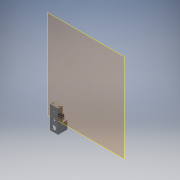
# Autodesk Inventor part: Xendmotorside
Saved by Autodesk Inventor 2016 (Build 200138000, 138)
## iProperties
Created: 2016-05-27
Part Number: Xendmotorside
Material: Generic
Document SubType Name: Modeling
Designer: Scott
Density: 1 g/cm^3
Appearance: Default
Author: Scott
Autodesk Inventor part; units mm, degrees
ref_plane "YZ Plane" through (0, 0, 0) normal (1, 0, 0) x (0, 1, 0)
ref_plane "XZ Plane" through (0, 0, 0) normal (0, 1, 0) x (-1, 0, 0)
ref_plane "XY Plane" through (0, 0, 0) normal (0, 0, 1) x (1, 0, 0)
ref_plane "Work Plane1" through (0, 0, 0) normal (0, 0, 1) x (1, 0, 0)
sketch "Sketch1" plane through (0, 0, 0) normal (0, 0, 1) x (1, 0, 0)
  circle A0 centre (0, 0) radius 6.35 projected
  circle A1 centre (0.5752, -49.1016) radius 4 projected
  line L0 (-12.7, -22.86) -> (12.7, -22.86)
  line L1 (12.7, -22.86) -> (12.7, 22.86)
  line L2 (12.7, 22.86) -> (-12.7, 22.86)
  line L3 (-12.7, 22.86) -> (-12.7, -22.86)
  line L4 (-12.7, -22.86) -> (12.7, 22.86) construction
  line L5 (12.7, -22.86) -> (-12.7, 22.86) construction
  line L6 (12.7, 22.86) -> (-12.7, 22.86)
  line L7 (-12.7, 22.86) -> (-12.7, -66.04)
  line L8 (-12.7, -66.04) -> (12.7, -66.04)
  line L9 (12.7, -66.04) -> (12.7, 22.86)
  point P0 (0, 0)
  dimension "d0" = 25.4
  dimension "d1" = 45.72
  dimension "d2" = 88.9
  constraints: 20 end point, 4 parallel, 2 horizontal, 2 midpoint, 2 perpendicular
  measures "d0" distance of L2.end L1.end
  measures "d1" distance of L1.end L0.end
  measures "d2" distance of L7.end L6.end
extrude "Extrusion1" add sketch "Sketch1" along normal blind 2.54
sketch "Sketch2" plane through (0, 0, 2.54) normal (0, 0, 1) x (1, 0, 0)
  circle A0 centre (0, 0) radius 6.35 projected
  circle A1 centre (0.5752, -49.1016) radius 4 projected
  line L0 (12.7, 22.86) -> (-12.7, 22.86) projected
  line L1 (-12.7, 22.86) -> (-12.7, -66.04) projected
  line L2 (-12.7, -66.04) -> (12.7, -66.04) projected
  line L3 (12.7, -66.04) -> (12.7, 22.86) projected
  circle A2 centre (0, 0) radius 7.62
  line L4 (0, 0) -> (0, -12.7)
  circle A3 centre (0, -12.7) radius 2.54
  line L5 (0, 0) -> (0, 12.7)
  circle A4 centre (0, 12.7) radius 2.54
  circle A5 centre (0.5752, -49.1016) radius 4 projected
  circle A6 centre (0.5752, -49.1016) radius 5
  point P0 (0, 0)
  dimension "d5" = 15.24
  dimension "d6" = 12.7
  dimension "d7" = 5.08
  dimension "d8" = 12.7
  dimension "d9" = 5.08
  dimension "d10" = 10
  constraints: 4 centre point, 4 coincident, 4 end point, 2 vertical
  measures "d5" diameter of A2
  measures "d6" distance of L4.start L4.end
  measures "d7" diameter of A3
  measures "d8" distance of L4.start L5.end
  measures "d9" diameter of A4
  measures "d10" diameter of A6
extrude "Extrusion2" cut sketch "Sketch2" against normal blind 2.54 contours A0 L4 L5 | A0 L5 A2 L4 | L5 L4 A0 | A0 L4 A2 L5 | A3 | A4 | A6
sketch "Sketch3" plane through (0, 0, 0) normal (0, 0, -1) x (-1, 0, 0)
  circle A0 centre (0, 0) radius 7.62 projected
  circle A1 centre (0, 12.7) radius 2.54 projected
  circle A2 centre (0, -12.7) radius 2.54 projected
  circle A3 centre (-0.5752, -49.1016) radius 5 projected
  line L0 (-12.7, 22.86) -> (12.7, 22.86) projected
  line L1 (-12.7, -66.04) -> (-12.7, 22.86) projected
  line L2 (12.7, -66.04) -> (-12.7, -66.04) projected
  line L3 (12.7, 22.86) -> (12.7, -66.04) projected
  line L4 (10.16, 19.05) -> (-10.16, 19.05)
  line L5 (-10.16, 19.05) -> (-10.16, -19.05)
  line L6 (-10.16, -19.05) -> (10.16, -19.05)
  line L7 (10.16, -19.05) -> (10.16, 19.05)
  circle A4 centre (0, 0) radius 7.62 projected
  line L8 (10.16, 19.05) -> (-10.16, -19.05) construction
  line L9 (-10.16, 19.05) -> (10.16, -19.05) construction
  point P0 (0, 0)
  dimension "d13" = 20.32
  dimension "d14" = 38.1
  constraints: 12 end point, 2 midpoint, 2 parallel, 1 horizontal, 1 perpendicular
  measures "d13" distance of L6.end L5.end
  measures "d14" distance of L5.end L4.end
extrude "Extrusion3" add sketch "Sketch3" along normal blind 25.4 contours L0 L3 L2 L1
sketch "Sketch4" plane through (0, 0, 2.54) normal (0, 0, 1) x (1, 0, 0)
  line L0 (-12.7, -66.04) -> (12.7, -66.04) projected
  line L1 (0, -66.04) -> (0, -90.8431)
  line L2 (24.81, -115.6589) -> (-24.81, -115.6589)
  line L3 (-24.81, -115.6589) -> (-24.81, -66.0273)
  line L4 (-24.81, -66.0273) -> (24.81, -66.0273)
  line L5 (24.81, -66.0273) -> (24.81, -115.6589)
  line L6 (24.81, -115.6589) -> (-24.81, -66.0273) construction
  line L7 (-24.81, -115.6589) -> (24.81, -66.0273) construction
  circle A0 centre (0, -90.8431) radius 12.5
  line L8 (0, -90.8431) -> (-15.5, -90.8431)
  line L9 (-15.5, -90.8431) -> (-15.5, -75.3431)
  circle A1 centre (-15.5, -75.3431) radius 2
  circle A2 centre (-15.5, -106.3467) radius 2
  circle A3 centre (15.5, -106.3467) radius 2
  circle A4 centre (15.5, -75.3395) radius 2
  point P0 (0, 0)
  dimension "d17" = 24.8031
  dimension "d18" = 49.62
  dimension "d19" = 49.6316
  dimension "d20" = 25
  dimension "d21" = 15.5
  dimension "d22" = 15.5
  dimension "d23" = 4
  dimension "d24" = 4
  dimension "d25" = 4
  dimension "d26" = 4
  constraints: 18 end point, 5 centre point, 3 midpoint, 3 point on line, 2 coincident, 2 horizontal, 2 parallel, 2 vertical, 1 perpendicular
  measures "d17" distance of L1.start L1.end
  measures "d18" distance of L3.end L4.end
  measures "d19" distance of L2.end L3.end
  measures "d20" diameter of A0
  measures "d21" distance of L8.start L8.end
  measures "d22" distance of L8.end L9.end
  measures "d23" diameter of A1
  measures "d24" diameter of A2
  measures "d25" diameter of A3
  measures "d26" diameter of A4
extrude "Extrusion4" add sketch "Sketch4" against normal blind 5.08
sketch "Sketch5" plane through (0, 0, -2.54) normal (0, 0, -1) x (-1, 0, 0)
  circle A0 centre (0, -90.8431) radius 12.5 projected
  circle A1 centre (-15.5, -75.3395) radius 2 projected
  circle A2 centre (-15.5, -106.3467) radius 2 projected
  circle A3 centre (15.5, -106.3467) radius 2 projected
  circle A4 centre (15.5, -75.3431) radius 2 projected
  line L0 (-12.7, -66.0273) -> (-12.7, 22.86) projected
  line L1 (-12.7, 22.86) -> (12.7, 22.86) projected
  line L2 (12.7, 22.86) -> (12.7, -66.0273) projected
  line L3 (24.81, -66.0273) -> (12.7, -66.0273) projected
  line L4 (24.81, -115.6589) -> (24.81, -66.0273) projected
  line L5 (-24.81, -115.6589) -> (24.81, -115.6589) projected
  line L6 (-24.81, -66.0273) -> (-24.81, -115.6589) projected
  line L7 (-12.7, -66.0273) -> (-24.81, -66.0273) projected
  circle A5 centre (0, 0) radius 7.62 projected
  circle A6 centre (0, 12.7) radius 2.54 projected
  circle A7 centre (0, -12.7) radius 2.54 projected
  circle A8 centre (-0.5752, -49.1016) radius 5 projected
  line L8 (24.81, -66.0273) -> (12.7, -66.0273) projected
  line L9 (-24.81, -115.6589) -> (24.81, -115.6589)
  line L10 (24.81, -115.6589) -> (24.81, -66.0273)
  line L11 (24.81, -66.0273) -> (-24.81, -66.0273)
  line L12 (-24.81, -66.0273) -> (-24.81, -115.6589)
  line L13 (-24.81, -115.6589) -> (24.81, -66.0273) construction
  line L14 (24.81, -115.6589) -> (-24.81, -66.0273) construction
  line L15 (-22, -112.8431) -> (22, -112.8431)
  line L16 (22, -112.8431) -> (22, -68.8431)
  line L17 (22, -68.8431) -> (-22, -68.8431)
  line L18 (-22, -68.8431) -> (-22, -112.8431)
  line L19 (-22, -112.8431) -> (22, -68.8431) construction
  line L20 (22, -112.8431) -> (-22, -68.8431) construction
  point P0 (0, 0)
  dimension "d29" = 44
  dimension "d30" = 44
  constraints: 24 end point, 4 midpoint, 4 parallel, 2 horizontal, 2 perpendicular
  measures "d29" distance of L17.end L16.end
  measures "d30" distance of L16.end L15.end
extrude "Extrusion5" add sketch "Sketch5" along normal blind 50.8 contours L11 L3 L4 L5 L6 L7
sketch "Sketch6" plane through (0, 0, -53.34) normal (0, 0, -1) x (-1, 0, 0)
  line L0 (22, -68.8431) -> (22, -112.8431) projected
  line L1 (22, -112.8431) -> (50.6459, -112.8431)
  line L2 (50.6459, -112.8431) -> (50.6459, -68.8431)
  line L3 (50.6459, -68.8431) -> (22, -68.8431)
  line L4 (22, -68.8431) -> (22, -112.8431)
  point P0 (0, 0)
  constraints: 8 end point, 2 parallel, 1 horizontal, 1 perpendicular
extrude "Extrusion6" cut sketch "Sketch6" against normal blind 50.8
chamfer "Chamfer1" distance 44.45 angle 45 1 edges at (-24.81, -114.251, -53.34)
sketch "Sketch7" plane through (12.7, -66.0273, 2.54) normal (0, 1, 0) x (1, 0, 0)
  line L0 (-25.4, 27.94) -> (-25.4, 0) projected
  line L1 (0, 27.94) -> (-25.4, 27.94) projected
  line L2 (0, 0) -> (0, 27.94) projected
  line L3 (0, 0) -> (12.11, 0) projected
  line L4 (12.11, 0) -> (12.11, 55.88) projected
  line L5 (-37.51, 55.88) -> (12.11, 55.88) projected
  line L6 (-37.51, 0) -> (-37.51, 55.88) projected
  line L7 (-37.51, 0) -> (-25.4, 0) projected
  line L8 (6.055, 0) -> (6.055, 12.7)
  circle A0 centre (6.055, 12.7) radius 4
  circle A1 centre (-31.455, 12.7) radius 4
  line L9 (0, 27.94) -> (12.11, 27.94)
  line L10 (12.11, 0) -> (12.11, 55.88) projected
  line L11 (-25.4, 27.94) -> (-37.51, 27.94)
  line L12 (-37.51, 55.88) -> (-37.51, 5.08) projected
  point P0 (-12.7, 2.54)
  dimension "d38" = 12.7
  dimension "d39" = 8
  dimension "d40" = 8
  constraints: 6 end point, 2 centre point, 2 midpoint, 2 point on line, 1 coincident, 1 vertical
  measures "d38" distance of L8.start L8.end
  measures "d39" diameter of A0
  measures "d40" diameter of A1
extrude "Extrusion7" add sketch "Sketch7" along normal up to surface (88.8873 mm away) contours L0 L7 L6 L11 | L9 L4 L3 L2
sketch "Sketch8" plane through (0, 0, -25.4) normal (0, 0, -1) x (-1, 0, 0)
  line L0 (24.81, -66.0273) -> (-24.81, -66.0273) projected
  line L1 (24.81, -66.0273) -> (24.81, 22.86) projected
  line L2 (24.81, 22.86) -> (-24.81, 22.86) projected
  line L3 (-24.81, -66.0273) -> (-24.81, 22.86) projected
  line L4 (10.16, 19.05) -> (10.16, -19.05) projected
  line L5 (10.16, -19.05) -> (-10.16, -19.05) projected
  line L6 (-10.16, -19.05) -> (-10.16, 19.05) projected
  line L7 (-10.16, 19.05) -> (10.16, 19.05) projected
  circle A0 centre (-0.5752, -49.1016) radius 5 projected
  circle A1 centre (-0.5752, -49.1016) radius 12.7
  point P0 (0, 0)
  dimension "d43" = 25.4
  constraints: 1 centre point, 1 coincident
  measures "d43" diameter of A1
extrude "Extrusion8" add sketch "Sketch8" along normal blind 12.7 contours A1
sketch "Sketch9" plane through (0.5752, -49.1016, -38.1) normal (0, 0, -1) x (-1, 0, 0)
  circle A0 centre (0, 0) radius 12.7 projected
  line L0 (25.3852, -16.9257) -> (-24.2348, -16.9257) projected
  line L1 (25.3852, -16.9257) -> (25.3852, 71.9616) projected
  line L2 (25.3852, 71.9616) -> (-24.2348, 71.9616) projected
  line L3 (-24.2348, -16.9257) -> (-24.2348, 71.9616) projected
  line L4 (10.7352, 68.1516) -> (10.7352, 30.0516) projected
  line L5 (10.7352, 30.0516) -> (-9.5848, 30.0516) projected
  line L6 (-9.5848, 30.0516) -> (-9.5848, 68.1516) projected
  line L7 (-9.5848, 68.1516) -> (10.7352, 68.1516) projected
  line L8 (-12.7, 0) -> (-12.7, -16.9257)
  line L9 (25.3852, -16.9257) -> (-24.2348, -16.9257) projected
  circle A1 centre (0, 0) radius 12.7 projected
  line L10 (12.7, 0) -> (12.7, -16.9257)
  line L11 (12.7, -16.9257) -> (-12.7, -16.9257)
  point P0 (0.5752, 49.1016)
  constraints: 6 end point, 2 perpendicular, 2 point on circle, 2 point on line, 1 collinear, 1 horizontal alignment, 1 vertical, 1 other
extrude "Extrusion9" add sketch "Sketch9" against normal up to surface (12.7 mm away) contours L10 L0 L8 A0
sketch "Sketch10" plane through (0, 0, -38.1) normal (0, 0, -1) x (-1, 0, 0)
  circle A0 centre (-0.5752, -49.1016) radius 5 projected
  circle A1 centre (-0.5752, -49.1016) radius 7.5
  point P0 (0, 0)
  dimension "d48" = 15
  constraints: 1 centre point, 1 coincident
  measures "d48" diameter of A1
sketch "Sketch11" plane through (0, 0, 2.54) normal (0, 0, 1) x (1, 0, 0)
  circle A0 centre (0.5752, -49.1016) radius 5 projected
  circle A1 centre (0.5752, -49.1016) radius 7.5
  point P0 (0, 0)
  dimension "d49" = 15
  constraints: 1 centre point, 1 coincident
  measures "d49" diameter of A1
extrude "Extrusion10" cut sketch "Sketch11" against normal blind 24
sketch "Sketch12" plane through (0, 0, -38.1) normal (0, 0, -1) x (-1, 0, 0)
  circle A0 centre (-0.5752, -49.1016) radius 5 projected
  arc A1 (12.1248, -49.1016) -> (-13.2752, -49.1016) centre (-0.5752, -49.1016) ccw projected
  line L0 (-13.2752, -49.1016) -> (-13.2752, -66.0273) projected
  line L1 (12.1248, -66.0273) -> (-13.2752, -66.0273) projected
  line L2 (12.1248, -66.0273) -> (12.1248, -49.1016) projected
  point P0 (0, 0)
extrude "Extrusion11" add sketch "Sketch12" along normal blind 8.89
sketch "Sketch13" plane through (0, 0, -46.99) normal (0, 0, -1) x (-1, 0, 0)
  circle A0 centre (-0.5752, -49.1016) radius 5 projected
  arc A1 (12.1248, -49.1016) -> (-13.2752, -49.1016) centre (-0.5752, -49.1016) ccw projected
  line L0 (-13.2752, -49.1016) -> (-13.2752, -66.0273) projected
  line L1 (12.1248, -66.0273) -> (-13.2752, -66.0273) projected
  line L2 (12.1248, -66.0273) -> (12.1248, -49.1016) projected
  circle A2 centre (-0.5752, -49.1016) radius 7.5
  point P0 (0, 0)
  dimension "d54" = 15
  constraints: 1 centre point, 1 coincident
  measures "d54" diameter of A2
extrude "Extrusion12" cut sketch "Sketch13" against normal blind 24 contours A2
sketch "Sketch14" plane through (24.81, -115.6589, 2.54) normal (1, 0, 0) x (0, 0, -1)
  spline S0 degree 2 poles (6.6012, 5.0914) (10.3495, 6.6696) (13.0128, 10.9605) knots 0 0 0 1 1 1
  spline S1 degree 2 poles (13.0128, 10.9605) (14.6897, 14.0677) (14.6897, 14.6102) knots 0 0 0 1 1 1
  line L0 (14.6897, 14.6102) -> (14.2952, 14.6102)
  spline S2 degree 2 poles (14.2952, 14.6102) (13.0128, 14.6102) (8.8206, 7.0642) knots 0 0 0 1 1 1
  line L1 (8.8206, 7.0642) -> (8.722, 7.0642)
  line L2 (8.722, 7.0642) -> (8.722, 7.3108)
  spline S3 degree 2 poles (8.722, 7.3108) (11.3359, 12.7854) (11.3359, 16.583) knots 0 0 0 1 1 1
  spline S4 degree 2 poles (11.3359, 16.583) (11.3359, 18.0133) (9.1165, 23.192) knots 0 0 0 1 1 1
  spline S5 degree 2 poles (9.1165, 23.192) (8.574, 25.3621) (8.574, 26.743) knots 0 0 0 1 1 1
  line L3 (8.574, 26.743) -> (8.574, 28.272)
  spline S6 degree 2 poles (8.574, 28.272) (8.574, 35.67) (12.6183, 45.8793) knots 0 0 0 1 1 1
  line L4 (12.6183, 45.8793) -> (12.8649, 46.9151)
  line L5 (12.8649, 46.9151) -> (13.1608, 46.9151)
  line L6 (13.1608, 46.9151) -> (13.1608, 45.0902)
  spline S7 degree 2 poles (13.1608, 45.0902) (13.2594, 42.0817) (13.654, 42.0817) knots 0 0 0 1 1 1
  spline S8 degree 2 poles (13.654, 42.0817) (17.4517, 43.4133) (20.0656, 43.4133) knots 0 0 0 1 1 1
  spline S9 degree 2 poles (20.0656, 43.4133) (24.9484, 43.4133) (30.9654, 38.7279) knots 0 0 0 1 1 1
  spline S10 degree 2 poles (30.9654, 38.7279) (37.0812, 31.6257) (38.9554, 22.3042) knots 0 0 0 1 1 1
  spline S11 degree 2 poles (38.9554, 22.3042) (39.4486, 19.4929) (39.4486, 14.7582) knots 0 0 0 1 1 1
  line L7 (39.4486, 14.7582) -> (39.4486, 13.969)
  spline S12 degree 2 poles (39.4486, 13.969) (41.8159, 7.5574) (46.8466, 5.0914) knots 0 0 0 1 1 1
  spline S13 degree 2 poles (46.8466, 5.0914) (47.2412, 5.0914) (47.2412, 4.8448) knots 0 0 0 1 1 1
  line L8 (47.2412, 4.8448) -> (46.452, 4.5982)
  line L9 (46.452, 4.5982) -> (46.3534, 4.5982)
  spline S14 degree 2 poles (46.3534, 4.5982) (44.4299, 4.5982) (39.5472, 9.7768) knots 0 0 0 1 1 1
  line L10 (39.5472, 9.7768) -> (39.5472, 9.6782)
  line L11 (39.5472, 9.6782) -> (39.6952, 7.5574)
  line L12 (39.6952, 7.5574) -> (39.6952, 7.3108)
  line L13 (39.6952, 7.3108) -> (39.4486, 7.3108)
  spline S15 degree 2 poles (39.4486, 7.3108) (38.1169, 12.7854) (35.6509, 14.6102) knots 0 0 0 1 1 1
  spline S16 degree 2 poles (35.6509, 14.6102) (35.6509, 14.8568) (34.3686, 14.8568) knots 0 0 0 1 1 1
  line L14 (34.3686, 14.8568) -> (31.3107, 14.8568)
  line L15 (31.3107, 14.8568) -> (31.3107, 11.7496)
  spline S17 degree 2 poles (31.3107, 11.7496) (31.3107, 11.3057) (33.2342, 10.9605) knots 0 0 0 1 1 1
  line L16 (33.2342, 10.9605) -> (33.2342, 10.7139)
  line L17 (33.2342, 10.7139) -> (26.0334, 10.7139)
  line L18 (26.0334, 10.7139) -> (26.0334, 10.9605)
  spline S18 degree 2 poles (26.0334, 10.9605) (26.6746, 10.9605) (27.3157, 12.1442) knots 0 0 0 1 1 1
  line L19 (27.3157, 12.1442) -> (27.3157, 14.8568)
  line L20 (27.3157, 14.8568) -> (21.5946, 14.8568)
  line L21 (21.5946, 14.8568) -> (21.348, 15.1527)
  line L22 (21.348, 15.1527) -> (21.5946, 16.2871)
  spline S19 degree 2 poles (21.5946, 16.2871) (21.2493, 17.8654) (20.0656, 17.8654) knots 0 0 0 1 1 1
  spline S20 degree 2 poles (20.0656, 17.8654) (18.3887, 17.8654) (17.6983, 14.3636) knots 0 0 0 1 1 1
  spline S21 degree 2 poles (17.6983, 14.3636) (16.12, 11.6017) (10.9414, 6.5217) knots 0 0 0 1 1 1
  spline S22 degree 2 poles (10.9414, 6.5217) (8.5247, 4.7461) (7.5383, 4.7461) knots 0 0 0 1 1 1
  line L23 (7.5383, 4.7461) -> (7.3903, 4.7461)
  spline S23 degree 2 poles (7.3903, 4.7461) (6.6012, 4.8448) (6.6012, 5.0914) knots 0 0 0 1 1 1
  line L24 (17.6983, 20.6273) -> (27.3157, 20.6273)
  spline S24 degree 2 poles (27.3157, 20.6273) (27.3157, 22.4522) (25.0963, 23.0933) knots 0 0 0 1 1 1
  spline S25 degree 2 poles (25.0963, 23.0933) (24.7511, 23.0933) (24.7511, 23.3399) knots 0 0 0 1 1 1
  line L25 (24.7511, 23.3399) -> (24.7511, 23.4879)
  line L26 (24.7511, 23.4879) -> (33.9247, 23.4879)
  spline S26 degree 2 poles (33.9247, 23.4879) (33.7274, 22.9947) (31.7053, 22.3042) knots 0 0 0 1 1 1
  line L27 (31.7053, 22.3042) -> (31.3107, 20.6273)
  line L28 (31.3107, 20.6273) -> (34.6152, 20.6273)
  spline S27 degree 2 poles (34.6152, 20.6273) (34.2206, 23.8331) (33.3328, 26.3485) knots 0 0 0 1 1 1
  spline S28 degree 2 poles (33.3328, 26.3485) (32.2478, 28.9131) (29.9297, 31.2805) knots 0 0 0 1 1 1
  line L29 (29.9297, 31.2805) -> (29.9297, 31.4285)
  line L30 (29.9297, 31.4285) -> (30.5709, 31.4285)
  spline S29 degree 2 poles (30.5709, 31.4285) (32.7903, 31.0832) (36.3414, 22.6988) knots 0 0 0 1 1 1
  line L31 (36.3414, 22.6988) -> (36.9825, 20.6273)
  spline S30 degree 2 poles (36.9825, 20.6273) (37.821, 20.6273) (38.0183, 21.7617) knots 0 0 0 1 1 1
  spline S31 degree 2 poles (38.0183, 21.7617) (35.7495, 30.0968) (30.3243, 33.8945) knots 0 0 0 1 1 1
  spline S32 degree 2 poles (30.3243, 33.8945) (26.132, 37.1496) (20.7068, 37.1496) knots 0 0 0 1 1 1
  spline S33 degree 2 poles (20.7068, 37.1496) (14.2952, 37.1496) (11.4346, 32.0696) knots 0 0 0 1 1 1
  spline S34 degree 2 poles (11.4346, 32.0696) (10.7934, 30.2448) (10.7934, 28.4199) knots 0 0 0 1 1 1
  spline S35 degree 2 poles (10.7934, 28.4199) (10.7934, 22.9947) (13.1608, 21.5151) knots 0 0 0 1 1 1
  spline S36 degree 2 poles (13.1608, 21.5151) (14.5911, 20.6273) (17.6983, 20.6273) knots 0 0 0 1 1 1
  point P0 (2.54, 115.6589)
  point P1 (6.6012, 7.5081)
  constraints: 1 other
extrude "Extrusion13" add sketch "Sketch14" along normal blind 1.27
sketch "Sketch16" plane through (0, 0, 2.54) normal (0, 0, 1) x (1, 0, 0)
  circle A0 centre (0.5752, -49.1016) radius 7.5 projected
  circle A1 centre (0, -90.8431) radius 12.5 projected
  circle A2 centre (15.5, -75.3395) radius 2 projected
  circle A3 centre (15.5, -106.3467) radius 2 projected
  circle A4 centre (-15.5, -106.3467) radius 2 projected
  circle A5 centre (-15.5, -75.3431) radius 2 projected
  line L0 (24.81, 22.86) -> (-24.81, 22.86) projected
  line L1 (-24.81, -115.6589) -> (-24.81, 22.86) projected
  line L2 (24.81, -115.6589) -> (-24.81, -115.6589) projected
  line L3 (24.81, -115.6589) -> (24.81, 22.86) projected
  circle A6 centre (0, 0) radius 7.62 projected
  circle A7 centre (0, 12.7) radius 2.54 projected
  circle A8 centre (0, -12.7) radius 2.54 projected
  arc A9 (-37.4082, 743.5284) -> (-37.4082, 731.1093) centre (-36.08, 737.3189) ccw projected
  line L4 (-24.81, 716.3555) -> (-24.81, 689.7) projected
  line L5 (28.62, 689.7) -> (-24.81, 689.7) projected
  line L6 (28.62, 828.2189) -> (-28.62, 828.2189) projected
  line L7 (-28.62, 828.2189) -> (-28.62, 772.2537) projected
  circle A10 centre (0, 799.0314) radius 2.54 projected
  circle A11 centre (-36.08, 737.3189) radius 2 projected
  circle A12 centre (0.5752, 761.6616) radius 7.5 projected
  circle A13 centre (0, 712.56) radius 7.62 projected
  circle A14 centre (0, 699.86) radius 2.54 projected
  circle A15 centre (0, 725.26) radius 2.54 projected
  line L8 (24.81, 22.86) -> (-24.81, 22.86) projected
  line L9 (24.81, 22.86) -> (28.62, 22.86)
  line L10 (28.62, 22.86) -> (28.62, -49.1016)
  line L11 (28.62, -49.1016) -> (24.81, -56.6016)
  line L12 (24.81, -66.0273) -> (24.81, 22.86) projected
  line L13 (-21.2845, -3.7955) -> (-46.08, -3.7955) projected
  line L14 (-26.08, 1) -> (-26.08, 21) projected
  line L15 (-46.08, 1) -> (-26.08, 1) projected
  line L16 (-46.08, 21) -> (-46.08, 1) projected
  line L17 (-26.08, 21) -> (-46.08, 21) projected
  line L18 (-24.81, -115.6589) -> (-24.81, 22.86) projected
  line L19 (-24.81, -3.7955) -> (-28.62, -3.7955)
  line L20 (-28.62, -3.7955) -> (-28.62, -49.1016)
  line L21 (-28.62, -49.1016) -> (-24.81, -54.7266)
  line L22 (-24.81, -66.0273) -> (-24.81, 22.86) projected
  arc A16 (-28.62, 772.2537) -> (-27.6419, 766.2281) centre (-9.57, 772.2537) ccw projected
  line L23 (-27.6419, 766.2281) -> (-26.9442, 764.1356) projected
  line L24 (-28.62, 761.6616) -> (-26.9442, 764.1356) projected
  line L25 (-28.62, 720.1655) -> (-28.62, 720.2426) projected
  line L26 (-28.62, 754.3951) -> (-28.62, 761.6616) projected
  line L27 (-28.62, 720.1655) -> (-24.81, 716.3555) projected
  line L28 (28.62, 689.7) -> (28.62, 725.7979) projected
  line L29 (29.89, 725.7979) -> (28.62, 725.7979) projected
  line L30 (29.89, 726.3679) -> (29.89, 725.7979) projected
  line L31 (28.62, 726.3679) -> (29.89, 726.3679) projected
  line L32 (28.62, 726.3679) -> (28.62, 828.2189) projected
  arc A17 (-37.4082, 743.5284) -> (-28.62, 754.3951) centre (-39.7325, 754.3951) ccw projected
  arc A18 (-28.62, 720.2426) -> (-37.4082, 731.1093) centre (-39.7325, 720.2426) ccw projected
  point P0 (0, 0)
  dimension "d61" = 3.81
  constraints: 12 end point, 5 point on line, 2 perpendicular, 1 horizontal
  measures "d61" distance of L19.start L19.end
extrude "Extrusion15" add sketch "Sketch16" against normal up to surface (27.94 mm away) contours L9 L10 L11 L3 | L1 L21 L20 L13
chamfer "Chamfer2" distance 3.81 angle 45 1 edges at (-28.62, -3.7955, -11.43)
body "Solid1"
